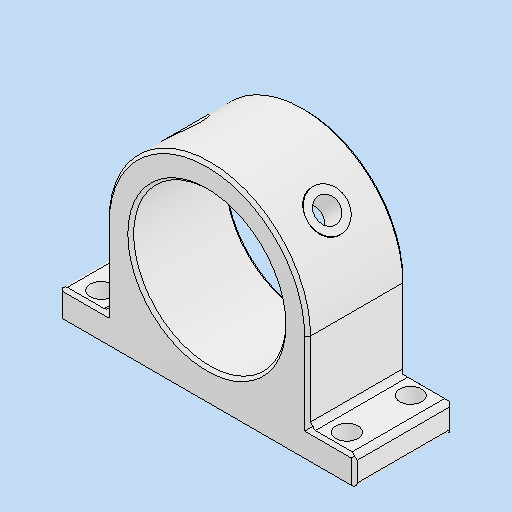
# Autodesk Inventor part: lens-clamp
Saved by Autodesk Inventor 2025 (Build 290162000, 162)
## iProperties
Created: 2025-06-06
Part Number: lens-clamp
Material: ABS Plastic
Document SubType Name: Modeling
Designer: kuzmin
Density: 1.06 g/cm^3
Appearance: Smooth - White
Author: kuzmin
Autodesk Inventor part; units mm, degrees
ref_plane "XZ Plane" through (0, 0, 0) normal (0, 1, 0) x (-1, 0, 0)
ref_plane "XY Plane" through (0, 0, 0) normal (0, 0, 1) x (1, 0, 0)
sketch "Sketch1" plane through (0, 0, 0) normal (0, 0, 1) x (1, 0, 0)
  circle A0 centre (0, 0) radius 15.5
  arc A1 (20.5, 0) -> (-20.5, 0) centre (0, 0) ccw
  line L0 (-30, -22.15) -> (30, -22.15)
  line L1 (20.5, 0) -> (20.5, -16.15)
  line L2 (20.5, -16.15) -> (30, -16.15)
  line L3 (30, -16.15) -> (30, -22.15)
  line L4 (-20.5, 0) -> (-20.5, -16.15)
  line L5 (-20.5, -16.15) -> (-30, -16.15)
  line L6 (-30, -16.15) -> (-30, -22.15)
  point P0 (0, -22.15)
  point P1 (0, -15.5)
  dimension "d0" = 31
  dimension "d1" = 60
  dimension "d4" = 6.65
  dimension "d18" = 6
  dimension "d35" = 41
  constraints: 14 end point, 3 perpendicular, 3 vertical alignment, 2 coincident, 2 point on circle, 2 point on line, 2 tangent, 1 centre point, 1 horizontal, 1 midpoint, 1 parallel, 1 vertical, 2 other
  measures "d1" distance of L0.start L0.end
  measures "d4" distance of point (0, -22.15) point (0, -15.5)
  measures "d18" distance of L5.end L0.start
  measures "d35" distance between parallel lines of L4 L1
extrude "Extrusion1" add sketch "Sketch1" along normal mid plane 20
sketch "Sketch4" plane through (20.5, -16.15, 10) normal (0, 1, 0) x (1, 0, 0)
  line L0 (4.5, 3.5) -> (-45.5, 3.5) construction
  line L1 (-45.5, 3.5) -> (-45.5, 16.5) construction
  line L2 (-45.5, 16.5) -> (4.5, 16.5) construction
  line L3 (4.5, 16.5) -> (4.5, 3.5) construction
  point P0 (-20.5, 10)
  point P1 (-20.5, 3.5)
  point P2 (-45.5, 10)
  dimension "d19" = 13
  dimension "d20" = 50
  constraints: 8 end point, 4 coincident, 2 midpoint, 2 parallel, 1 horizontal, 1 horizontal alignment, 1 perpendicular, 1 vertical alignment
  measures "d19" distance of L0.end L1.end
  measures "d20" distance of L0.start L0.end
hole "Hole2" at (25, -16.15, 6.5) at (-25, -16.15, 6.5) at (-25, -16.15, -6.5) at (25, -16.15, -6.5) direction (0, -1, 0) diameter 4.5 end through all
chamfer "Chamfer1" distance 0.6 angle 45 18 edges at (0, 20.5, -10) (20.5, -8.075, -10) (-20.5, -8.075, -10) (-15.5, 0, -10) (-25.25, -16.15, -10) (25.25, -16.15, -10) (30, -19.15, -10) (0, -22.15, -10) (-30, -19.15, -10) (0, 20.5, 10) (-20.5, -8.075, 10) (20.5, -8.075, 10) (-25.25, -16.15, 10) (-30, -19.15, 10) (0, -22.15, 10) (25.25, -16.15, 10) (30, -19.15, 10) (-15.5, 0, 10)
fillet "Fillet1" radius 1 6 edges at (30, -16.15, 0) (20.5, -16.15, 0) (30, -22.15, 0) (-30, -16.15, 0) (-30, -22.15, 0) (-20.5, -16.15, 0)
chamfer "Chamfer2" distance 0.4 angle 45 4 edges at (-25, -22.15, 4.25) (-25, -22.15, -8.75) (25, -22.15, 4.25) (25, -22.15, -8.75)
ref_plane "Work Plane2" through (0, 0, 0) normal (0.7071068, 0.7071068, 0) x (0, 0, 1)
ref_plane "Work Plane3" through (14.4957, 14.4957, 0) normal (0.7071068, 0.7071068, 0) x (0, 0, 1)
sketch "Sketch5" plane through (0, 0, 0) normal (0.7071068, 0.7071068, 0) x (0, 0, 1)
  point P0 (0, 0)
  point P1 (0, 0)
  constraints: 1 coincident
hole "Hole3" at (0, 0, 0) direction (0.7071068, 0.7071068, 0) diameter 4.9 end through all
sketch "Sketch6" plane through (14.4957, 14.4957, 0) normal (0.7071068, 0.7071068, 0) x (0, 0, 1)
  spline S0 degree 8 poles (-2.45, 0) (-2.45, -0.2861) (-2.4118, -0.5652) (-2.3387, -0.8315) (-2.2348, -1.0803) (-2.105, -1.3076) (-1.955, -1.5104) (-1.791, -1.6872) (-1.4416, -1.9952) (-1.2512, -2.1278) (-1.0523, -2.2366) (-0.8473, -2.3225) (-0.6382, -2.3864) (-0.4264, -2.4288) (-0.2133, -2.45) (0.2555, -2.45) (0.5106, -2.4196) (0.7634, -2.3588) (1.0117, -2.2671) (1.2529, -2.1432) (1.4831, -1.9854) (1.6972, -1.792) (2.0496, -1.3661) (2.2007, -1.1362) (2.3279, -0.8755) (2.421, -0.5902) (2.4734, -0.2891) (2.482, 0.0179) (2.4472, 0.3204) (2.3252, 0.7957) (2.2606, 0.9778) (2.1797, 1.1538) (2.0833, 1.3221) (1.9721, 1.481) (1.8472, 1.6291) (1.7099, 1.7651) (1.3986, 2.0227) (1.2222, 2.1415) (1.0343, 2.2427) (0.837, 2.3249) (0.6326, 2.3873) (0.4233, 2.4291) (0.2117, 2.45) (-0.2133, 2.45) (-0.4264, 2.4288) (-0.6382, 2.3864) (-0.8473, 2.3225) (-1.0523, 2.2366) (-1.2512, 2.1278) (-1.4416, 1.9952) (-1.7909, 1.6873) (-1.9549, 1.5105) (-2.105, 1.3076) (-2.2349, 1.0802) (-2.3388, 0.8314) (-2.4119, 0.565) (-2.45, 0.2859) (-2.45, 0) knots 0 0 0 0 0 0 0 0 0 0.137165 0.137165 0.137165 0.137165 0.137165 0.137165 0.137165 0.280572 0.280572 0.280572 0.280572 0.280572 0.280572 0.280572 0.452351 0.452351 0.452351 0.452351 0.452351 0.452351 0.452351 0.598232 0.598232 0.598232 0.598232 0.598232 0.598232 0.598232 0.692362 0.692362 0.692362 0.692362 0.692362 0.692362 0.692362 0.795904 0.795904 0.795904 0.795904 0.795904 0.795904 0.795904 0.900244 0.900244 0.900244 0.900244 0.900244 0.900244 0.900244 1 1 1 1 1 1 1 1 1 projected
  circle A0 centre (0, 0) radius 4
  dimension "d47" = 8
  constraints: 1 centre point, 1 coincident, 1 other
  measures "d47" diameter of A0
extrude "Extrusion2" add sketch "Sketch6" against normal up to surface
pattern_circular "Circular Pattern1" count 2 over 90 about axis through (0, 0, 0) along (0, 0, 1) of "Hole3", "Extrusion2"
body "Solid1"
